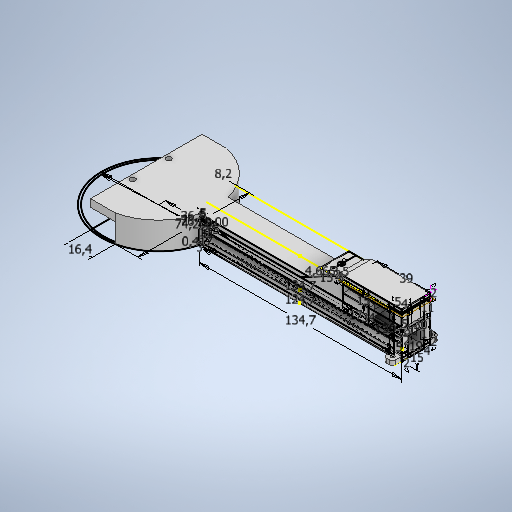
# Autodesk Inventor part: new_extrad_system
Saved by Autodesk Inventor 2025 (Build 290162000, 162)
## iProperties
Created: 2026-09-06
Part Number: new_extrad_system
Material: Типовые
Document SubType Name: Modeling
Designer: Leva
Density: 1 g/cm^3
Appearance: По умолчанию
Author: Leva
Autodesk Inventor part; units mm, degrees
ref_plane "YZ Plane" through (0, 0, 0) normal (1, 0, 0) x (0, 1, 0)
ref_plane "XZ Plane" through (0, 0, 0) normal (0, 1, 0) x (-1, 0, 0)
ref_plane "XY Plane" through (0, 0, 0) normal (0, 0, 1) x (1, 0, 0)
sketch "Эскиз1" plane through (0, 0, 0) normal (0, 0, 1) x (1, 0, 0)
  line L0 (-67.35, 7.5) -> (67.35, 7.5)
  line L1 (67.35, 7.5) -> (67.35, -7.5)
  line L2 (67.35, -7.5) -> (-67.35, -7.5)
  line L3 (-67.35, -7.5) -> (-67.35, 7.5)
  line L4 (-67.35, 7.5) -> (67.35, -7.5) construction
  line L5 (67.35, 7.5) -> (-67.35, -7.5) construction
  line L6 (-62.35, 2.5) -> (62.35, 2.5)
  line L7 (62.35, 2.5) -> (62.35, -2.5)
  line L8 (62.35, -2.5) -> (-62.35, -2.5)
  line L9 (-62.35, -2.5) -> (-62.35, 2.5)
  line L10 (-62.35, 2.5) -> (62.35, -2.5) construction
  line L11 (62.35, 2.5) -> (-62.35, -2.5) construction
  line L12 (-67.35, -7.5) -> (67.35, -7.5)
  line L13 (67.35, -7.5) -> (67.35, -5.5)
  line L14 (67.35, -5.5) -> (-67.35, -5.5)
  line L15 (-67.35, -5.5) -> (-67.35, -7.5)
  line L16 (-67.35, 7.5) -> (67.35, 7.5)
  line L17 (67.35, 7.5) -> (67.35, 5.5)
  line L18 (67.35, 5.5) -> (-67.35, 5.5)
  line L19 (-67.35, 5.5) -> (-67.35, 7.5)
  line L20 (67.35, -7.5) -> (62.35, -7.5)
  line L21 (62.35, -7.5) -> (62.35, 22.5)
  line L22 (62.35, 22.5) -> (67.35, 22.5)
  line L23 (67.35, 22.5) -> (67.35, -7.5)
  line L24 (62.35, 22.5) -> (45.35, 22.5)
  line L25 (45.35, 22.5) -> (45.35, 7.5)
  line L26 (45.35, 7.5) -> (62.35, 7.5)
  line L27 (62.35, 7.5) -> (62.35, 22.5)
  line L28 (45.35, 22.5) -> (28.35, 22.5)
  line L29 (28.35, 22.5) -> (28.35, 7.5)
  line L30 (28.35, 7.5) -> (45.35, 7.5)
  line L31 (45.35, 7.5) -> (45.35, 22.5)
  line L32 (67.35, 22.5) -> (28.35, 22.5)
  line L33 (28.35, 22.5) -> (28.35, 20.5)
  line L34 (28.35, 20.5) -> (67.35, 20.5)
  line L35 (67.35, 20.5) -> (67.35, 22.5)
  line L36 (28.35, 17.5) -> (62.35, 17.5)
  line L37 (62.35, 17.5) -> (62.35, 12.5)
  line L38 (62.35, 12.5) -> (28.35, 12.5)
  line L39 (28.35, 12.5) -> (28.35, 17.5)
  line L40 (28.35, 22.5) -> (0, 7.5)
  line L41 (-62.35, -2.5) -> (-67.35, -7.5)
  line L42 (-67.35, 5.5) -> (-62.35, 5.5)
  line L43 (-62.35, 5.5) -> (-62.35, 10.5)
  line L44 (-62.35, 10.5) -> (-67.35, 10.5)
  line L45 (-67.35, 10.5) -> (-67.35, 5.5)
  line L46 (-62.35, 10.5) -> (-67.35, 5.5) construction
  circle A0 centre (-64.85, 8) radius 1.25
  line L47 (-62.35, 10.5) -> (-48.6126, 5.5)
  line L48 (-62.35, 10.5) -> (-47.731, 10.5) construction
  line L49 (-67.35, 10.5) -> (-62.35, 10.5)
  line L50 (28.35, 22.5) -> (28.35, 19.5)
  line L51 (45.35, 7.5) -> (45.35, 2.5)
  line L52 (62.35, 12.5) -> (67.35, 12.5)
  line L53 (67.35, 12.5) -> (67.35, 7.5)
  line L54 (67.35, 7.5) -> (62.35, 7.5)
  line L55 (62.35, 7.5) -> (62.35, 12.5)
  line L56 (64.35, 11.5) -> (67.35, 11.5)
  line L57 (67.35, 11.5) -> (67.35, 8.5)
  line L58 (67.35, 8.5) -> (64.35, 8.5)
  line L59 (64.35, 8.5) -> (64.35, 11.5)
  line L60 (-62.35, 10.5) -> (5.67, 10.5)
  line L61 (28.35, 19.5) -> (38.35, 19.5) construction
  point P0 (0, 0)
  point P1 (62.35, 15)
  point P2 (45.35, 12.5)
  point P3 (28.35, 7.5)
  point P4 (-62.35, 7.5)
  point P5 (0, 7.5)
  point P6 (67.35, 10)
  point P7 (62.35, 7.5)
  point P8 (45.35, 17.5)
  point P9 (62.35, 5.5)
  point P10 (45.35, 5.5)
  point P11 (-63.7044, 7.5)
  point P12 (-65.9956, 7.5)
  dimension "d0" = 134.7
  dimension "d1" = 15
  dimension "d2" = 124.7
  dimension "d3" = 5
  dimension "d4" = 2
  dimension "d5" = 134.7
  dimension "d6" = 2
  dimension "d7" = 5
  dimension "d8" = 30
  dimension "d9" = 17
  dimension "d10" = 15
  dimension "d11" = 17
  dimension "d12" = 2
  dimension "d13" = 34
  dimension "d14" = 5
  dimension "d15" = 5
  dimension "d16" = 5
  dimension "d17" = 2.5
  dimension "d18" = 20
  dimension "d22" = 5
  dimension "d23" = 3
  dimension "d27" = 3
  dimension "d28" = 3
  constraints: 124 end point, 24 parallel, 15 horizontal, 13 perpendicular, 10 midpoint, 8 point on line, 1 centre point, 1 equal length
  measures "d0" distance of L1.end L2.end
  measures "d1" distance of L0.end L1.end
  measures "d2" distance of L7.end L8.end
  measures "d3" distance of L6.end L7.end
  measures "d4" distance of L13.end L12.end
  measures "d5" distance of L17.end L18.end
  measures "d6" distance of L16.end L17.end
  measures "d7" distance of L21.end L22.end
  measures "d8" distance of L20.end L21.end
  measures "d9" distance of L26.end L25.end
  measures "d10" distance of L25.end L24.end
  measures "d11" distance of L30.end L29.end
  measures "d12" distance of L33.end L32.end
  measures "d13" distance of L37.end L38.end
  measures "d14" distance of L36.end L37.end
  measures "d15" distance of L44.end L43.end
  measures "d16" distance of L43.end L42.end
  measures "d17" diameter of A0
  measures "d18" angle of L47 L48
  measures "d22" distance of L44.end L49.end
  measures "d23" distance of L32.end L50.end
  measures "d27" distance of L57.end L58.end
  measures "d28" distance of L56.end L57.end
extrude "Выдавливание1" add sketch "Эскиз1" against normal blind 19 contours L40 L29 L0 | L0 L51 L18 L47 | L0 L47 L60 L40 | L29 L38 L25 L0 | L47 L18 L43 L0 | L0 L43 L47 | L43 L18 L3 L0 A0 | L0 A0 L45 L44 L43 | L18 L51 L6 L9 L41 L14 L3 | L28 L25 L34 L29 | L21 L52 L23 L56 L59 L58 L0 | L0 L1 L18 L21 | L29 L34 L25 L36 | L24 L21 L34 L25 | L21 L34 L23 L52 | L18 L1 L14 L21 L7 | L25 L34 L21 L36 | L22 L23 L34 L21 | L14 L41 L3 | L1 L2 L21 L14 | L21 L14 L41 L8 | L41 L14 L21 L2
sketch "Эскиз2" plane through (67.35, -7.5, 0) normal (1, 0, 0) x (0, 0, -1)
  line L0 (0, 0) -> (19, 0)
  line L1 (19, 0) -> (19, 30)
  line L2 (19, 30) -> (0, 30)
  line L3 (0, 30) -> (0, 0)
  line L4 (0, 0) -> (4, 0)
  line L5 (4, 0) -> (4, 30)
  line L6 (4, 30) -> (0, 30)
  line L7 (0, 30) -> (0, 0)
  line L8 (19, 30) -> (15, 30)
  line L9 (15, 30) -> (15, 0)
  line L10 (15, 0) -> (19, 0)
  line L11 (19, 0) -> (19, 30)
  line L12 (0, 0) -> (19, 0)
  line L13 (19, 0) -> (19, 2)
  line L14 (19, 2) -> (0, 2)
  line L15 (0, 2) -> (0, 0)
  line L16 (4, 2) -> (15, 2)
  line L17 (15, 2) -> (15, 13)
  line L18 (15, 13) -> (4, 13)
  line L19 (4, 13) -> (4, 2)
  line L20 (0, 30) -> (19, 30)
  line L21 (19, 30) -> (19, 28)
  line L22 (19, 28) -> (0, 28)
  line L23 (0, 28) -> (0, 30)
  line L24 (4, 28) -> (15, 28)
  line L25 (15, 28) -> (15, 17)
  line L26 (15, 17) -> (4, 17)
  line L27 (4, 17) -> (4, 28)
  point P0 (0, 7.5)
  point P1 (15, 2)
  dimension "d29" = 4
  dimension "d30" = 30
  dimension "d31" = 4
  dimension "d32" = 30
  dimension "d33" = 19
  dimension "d34" = 2
  dimension "d35" = 11
  dimension "d36" = 2
  dimension "d37" = 11
  constraints: 56 end point, 14 parallel, 7 horizontal, 7 perpendicular, 7 point on line
  measures "d29" distance of L6.end L5.end
  measures "d30" distance of L5.end L4.end
  measures "d31" distance of L10.end L9.end
  measures "d32" distance of L9.end L8.end
  measures "d33" distance of L14.end L13.end
  measures "d34" distance of L13.end L12.end
  measures "d35" distance of L17.end L16.end
  measures "d36" distance of L20.end L21.end
  measures "d37" distance of L24.end L25.end
extrude "Выдавливание2" cut sketch "Эскиз2" against normal blind 134.7 contours L5 L18 L9 L14
extrude "Выдавливание3" cut sketch "Эскиз2" against normal blind 34 from surface at -5 contours L22 L9 L26 L5
sketch "Эскиз3" plane through (-67.35, -7.5, 0) normal (0, -1, 0) x (1, 0, 0)
  line L0 (0, -15) -> (0, -4) projected
  line L1 (0, -9.5) -> (-36.5, -9.5) construction
  circle A0 centre (-36.5, -9.5) radius 38
  circle A1 centre (-36.5, -9.5) radius 36.5
  line L2 (-36.5, -9.5) -> (-28.3, -9.5) construction
  line L3 (-28.3, -9.5) -> (-28.3, -46.6047) construction
  line L4 (-28.3, -46.6047) -> (-36.5, -46.6047) construction
  line L5 (-36.5, -46.6047) -> (-36.5, -9.5) construction
  line L6 (-28.3, -46.6047) -> (-28.3, 27.6047)
  line L7 (3, -15) -> (0, -15)
  line L8 (0, -15) -> (0, -4)
  line L9 (0, -4) -> (3, -4)
  line L10 (3, -4) -> (3, -15)
  line L11 (0, 0) -> (0, -19) projected
  line L12 (0, -15) -> (-0.417, -15)
  line L13 (-0.417, -15) -> (-0.417, -4)
  line L14 (-0.417, -4) -> (0, -4)
  line L15 (0, -4) -> (0, -15)
  line L16 (-44.7, -46.6045) -> (-28.3, -46.6045)
  line L17 (-28.3, -46.6045) -> (-28.3, 27.6045)
  line L18 (-28.3, 27.6045) -> (-44.7, 27.6045)
  line L19 (-44.7, 27.6045) -> (-44.7, -46.6045)
  point P0 (67.35, 0)
  point P1 (1.0999, -15)
  point P2 (1.0999, -4)
  point P3 (-0.4168, -4)
  point P4 (-28.3, 26.067)
  point P5 (-0.4168, -15)
  point P6 (-28.3, -45.067)
  point P7 (-28.3, -9.5)
  dimension "d42" = 36.5
  dimension "d43" = 76
  dimension "d44" = 73
  dimension "d45" = 8.2
  dimension "d46" = 3
  dimension "d47" = 11
  dimension "d48" = 0.417
  dimension "d49" = 11
  dimension "d59" = 16.4
  dimension "d60" = 74.209
  constraints: 36 end point, 8 parallel, 7 midpoint, 5 horizontal, 5 perpendicular, 2 centre point, 2 coincident, 2 point on circle
  measures "d42" distance of L1.start L1.end
  measures "d43" diameter of A0
  measures "d44" diameter of A1
  measures "d45" distance of L3.end L4.end
  measures "d46" distance of L8.end L9.end
  measures "d47" distance of L7.end L8.end
  measures "d48" distance of L13.end L14.end
  measures "d49" distance of L12.end L13.end
  measures "d59" distance of L18.end L17.end
  measures "d60" distance of L17.end L16.end
extrude "Выдавливание4" add sketch "Эскиз3" against normal blind 2 contours L12 A1 L0 | L7 A0 L6 A1 L12 | A1 L14 L0 | A1 L13 | A1 L6 L13 | L14 A1 L6 A0 L9
extrude "Выдавливание5" add sketch "Эскиз3" against normal blind 13 contours L7 A0 L6 A1 L12 | L14 A1 L6 A0 L9
extrude "Выдавливание6" add sketch "Эскиз3" against normal blind 5 from surface at -13 contours L12 A1 L0 | L0 L9 A0 L7 | L7 A0 L6 A1 L12 | A1 L14 L0 | A1 L13 | A1 L6 L13 | L14 A1 L6 A0 L9
extrude "Выдавливание7" add sketch "Эскиз3" along normal blind 5 from surface at -18 contours L16 L19 A1 L6 | A1 L19 L6 | A1 L19 L18 L6
ref_plane "РабПлоскость1" through (28.35, 19.5, 0) normal (0, 1, 0) x (1, 0, 0)
sketch "Эскиз5" plane through (28.35, 19.5, 0) normal (0, 1, 0) x (1, 0, 0)
  line L0 (39, 0) -> (39, 19) projected
  line L1 (-90.7, 19) -> (34, 19) projected
  line L2 (39, 0) -> (0, 0)
  line L3 (0, 0) -> (0, 19)
  line L4 (0, 19) -> (39, 19)
  line L5 (39, 19) -> (39, 0)
  line L6 (34, 0) -> (-90.7, 0) projected
  line L7 (0, 19) -> (-15, 19)
  line L8 (-15, 19) -> (-15, 0)
  line L9 (-15, 0) -> (0, 0)
  line L10 (0, 0) -> (0, 19)
  line L11 (-15, 19) -> (-10.335, 19)
  line L12 (-10.335, 19) -> (-10.335, 0)
  line L13 (-10.335, 0) -> (-15, 0)
  line L14 (-15, 0) -> (-15, 19)
  circle A0 centre (-10.335, 9.5) radius 1.75
  point P0 (-28.35, 0)
  dimension "d72" = 39
  dimension "d73" = 15
  dimension "d76" = 4.665
  dimension "d77" = 3.5
  constraints: 24 end point, 6 parallel, 3 horizontal, 3 perpendicular, 3 point on line, 1 centre point, 1 midpoint
  measures "d72" distance of L3.end L4.end
  measures "d73" distance of L9.end L8.end
  measures "d76" distance of L12.end L13.end
  measures "d77" diameter of A0
extrude "Выдавливание9" add sketch "Эскиз5" against normal blind 6 contours L6 L12 A0 L1 L3 | L6 L8 L1 L12 A0 | A0 L12 | L12 A0
extrude "Выдавливание10" cut sketch "Эскиз5" against normal blind 6 contours A0 L12 | L12 A0
sketch "Эскиз6" plane through (5.67, 10.5, 0) normal (0, 1, 0) x (1, 0, 0)
  line L0 (-114.72, 21.5) -> (-117.72, 21.5) construction
  line L1 (-117.72, 21.5) -> (-117.72, -2.5) construction
  line L2 (-117.72, -2.5) -> (-114.72, -2.5) construction
  line L3 (-114.72, -2.5) -> (-114.72, 21.5) construction
  line L4 (-117.72, -27.6045) -> (-117.72, 46.6045) projected
  circle A0 centre (-114.72, 21.5) radius 1.75
  circle A1 centre (-114.72, -2.5) radius 1.75
  point P0 (-5.67, 0)
  point P1 (-117.72, 9.5)
  dimension "d80" = 3
  dimension "d81" = 24
  dimension "d82" = 3.5
  dimension "d83" = 3.5
  constraints: 8 end point, 2 centre point, 2 coincident, 2 midpoint, 2 parallel, 1 horizontal, 1 perpendicular
  measures "d80" distance of L2.end L1.end
  measures "d81" distance of L1.end L0.end
  measures "d82" diameter of A0
  measures "d83" diameter of A1
extrude "Выдавливание11" cut sketch "Эскиз6" against normal blind 5
sketch "Эскиз7" plane through (67.35, -7.5, -19) normal (0, -1, 0) x (1, 0, 0)
  line L0 (0, 0) -> (-134.4067, 0) projected
  line L1 (0, 0) -> (-6, 0)
  line L2 (-6, 0) -> (-6, -6)
  line L3 (-6, -6) -> (0, -6)
  line L4 (0, -6) -> (0, 0)
  line L5 (-6, -3) -> (0, -3) construction
  line L6 (-3, 0) -> (-3, -6) construction
  circle A0 centre (-3, -3) radius 1.25
  line L7 (0, 19) -> (0, 0) construction
  line L8 (0, 9.5) -> (-10, 9.5) construction
  line L9 (0, 19) -> (-6, 19)
  line L10 (-6, 19) -> (-6, 25)
  line L11 (-6, 25) -> (0, 25)
  line L12 (0, 25) -> (0, 19)
  line L13 (-6, 22) -> (0, 22) construction
  line L14 (-3, 19) -> (-3, 25) construction
  circle A1 centre (-3, 22) radius 1.25
  point P0 (-67.35, 19)
  point P1 (-6, 0)
  dimension "d86" = 6
  dimension "d87" = 6
  dimension "d88" = 2.5
  dimension "d89" = 10
  constraints: 26 end point, 8 symmetric about line, 6 midpoint, 2 centre point, 2 horizontal, 2 parallel, 1 perpendicular, 1 other
  measures "d86" distance of L3.end L2.end
  measures "d87" distance of L2.end L1.end
  measures "d88" diameter of A0
  measures "d89" distance of L8.start L8.end
extrude "Выдавливание12" add sketch "Эскиз7" against normal blind 3
fillet "Сопряжение1" radius 2 6 edges at (61.35, -6, -25) (61.35, -6, -19) (61.35, -6, 6) (61.35, -6, 0) (67.35, -6, 6) (67.35, -6, -25)
